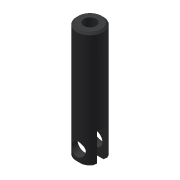
# Autodesk Inventor part: Pin Pressure
Saved by Autodesk Inventor 2022 Beta2 (Build 260130000, 130) ContinuousBuild 0
## iProperties
Created: 2006-01-31
Part Number: Pin Pressure
Document SubType Name: Modeling
Designer: landrews
Stock Number: Pin Pressure
Density: 1 g/cm^3
Material: Generic
Appearance: Generic
Author: landrews
Autodesk Inventor part; units mm, degrees
ref_plane "YZ Plane" through (0, 0, 0) normal (1, 0, 0) x (0, 1, 0)
ref_plane "XZ Plane" through (0, 0, 0) normal (0, 1, 0) x (-1, 0, 0)
ref_plane "XY Plane" through (0, 0, 0) normal (0, 0, 1) x (1, 0, 0)
sketch "Sketch1" plane through (0, 0, 0) normal (0, 0, 1) x (1, 0, 0)
  line L0 (0, 12) -> (0, -9) projected
  line L1 (-9, 0) -> (12, 0) projected
  circle A0 centre (0, 0) radius 7.5
  dimension "d0" = 15
  constraints: 2 point on line, 1 centre point
  measures "d0" diameter of A0
extrude "Extrusion1" add sketch "Sketch1" along normal blind 66
sketch "Sketch2" plane through (0, 0, 0) normal (1, 0, 0) x (0, 1, 0)
  line L0 (-3, -8.1335) -> (3, -8.1335)
  line L1 (3, -8.1335) -> (3, 18)
  line L2 (3, 18) -> (-3, 18)
  line L3 (-3, 18) -> (-3, -8.1335)
  line L4 (0, 88.24) -> (0, -15.5468) projected
  line L5 (-7.5, 0) -> (7.5, 0) projected
  dimension "d3" = 6
  dimension "d7" = 18
  constraints: 8 end point, 2 parallel, 1 horizontal, 1 perpendicular, 1 other
  measures "d3" distance of L0.start L0.end
  measures "d7" distance between parallel lines of L5 L2
extrude "Extrusion2" cut sketch "Sketch2" along normal through all both and the other way through all
sketch "Sketch3" plane through (0, 0, 0) normal (0, 1, 0) x (-1, 0, 0)
  line L0 (0, -6.6) -> (0, 85.8) projected
  circle A0 centre (0, 8) radius 4
  line L1 (-6.8739, 0) -> (6.8739, 0) projected
  dimension "d8" = 8
  dimension "d9" = 8
  constraints: 1 centre point, 1 point on line
  measures "d8" diameter of A0
  measures "d9" distance from line of L1 A0.centre
extrude "Extrusion3" cut sketch "Sketch3" along normal through all both and the other way through all
chamfer "Chamfer1" distance 2 angle 45 2 edges at (0, -7.5, 0) (0, 7.5, 0)
chamfer "Chamfer2" distance 1 angle 45 1 edges at (-7.5, 0, 66)
hole "Hole1" at (0, 0, 66) direction (0, 0, -1) diameter 6.917 depth 30 tip angle 118
body "Solid1"
